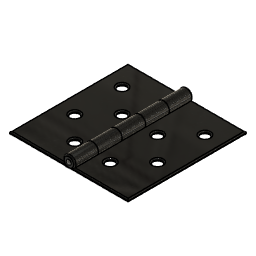
Hinge Joint (Autodesk Fusion 360 design; units mm, degrees)
Autodesk Fusion 360 part; units mm, degrees
sketch "Sketch1" plane through (0, 0, 0) normal (0, 1, 0) x (1, 0, 0)
  line L0 (0, 0) -> (50, 0)
  line L1 (50, 0) -> (50, 2.5)
  line L2 (50, 2.5) -> (0, 2.5)
  line L3 (0, 2.5) -> (0, 0)
  circle A0 centre (0, -2.5) radius 5
  circle A1 centre (0, -2.5) radius 2
  dimension "d1" = 50
  dimension "d2" = 2.5
  dimension "d3" = 10
  dimension "d4" = 4
  constraint horizontal L0
  constraint vertical L1
  constraint horizontal L2
  constraint vertical L3
  constraint coincident L0.start L3.end
  constraint coincident L2.end A0
  constraint concentric A0 A1
  measures "d1" distance of L0.start L0.end
  measures "d2" distance of L0.start L2.end
  measures "d3" diameter of A0
  measures "d4" diameter of A1
extrude "Extrude1" add sketch "Sketch1" along normal blind 100 contours L0 L1 L2 A0 makes body 1 in component "hinge1"
extrude "Extrude2" add sketch "Sketch1" along normal blind 20 contours L0 L3 A0 | L0 L3 A0 bodies 1 in component "hinge1"
pattern_linear "R-Pattern1" count 3 spacing 40 along (0, 1, 0) of "Extrude2" in component "hinge1"
extrude "Extrude1'" add sketch "Sketch1" along normal blind 100 separate body contours L0 L1 L2 A0 makes body 2 in component "hinge 2"
extrude "Extrude2'" add 1 faces at (3.5955, 20, 0.7685) along direction (0, 1, 0) blind 20 on bodies 1 bodies 2 in component "hinge 2"
extrude "Extrude3" add 1 faces at (-0.2982, 60, -1.4795) along direction (0, 1, 0) blind 20 on bodies 1 bodies 2 in component "hinge 2"
sketch "Sketch2" plane through (0, 0, 7.5) normal (0, 0, 1) x (-1, 0, 0)
  line L0 (-50, -100) -> (0, -100)
  line L1 (0, -100) -> (0, -80)
  line L2 (0, -80) -> (0, -60)
  line L3 (0, -60) -> (0, -40)
  line L4 (0, -40) -> (0, -20)
  line L5 (0, -20) -> (0, 0)
  line L6 (0, 0) -> (-50, 0)
  line L7 (-50, 0) -> (-50, -100)
  circle A0 centre (-35, -80) radius 3.75
  circle A1 centre (-35, -40) radius 3.75
  circle A2 centre (-15, -60) radius 3.75
  circle A3 centre (-15, -20) radius 3.75
  line L8 (0, 0) -> (-50, 0)
  dimension "d25" = 7.5
  dimension "d26" = 7.5
  dimension "d27" = 7.5
  dimension "d28" = 7.5
  dimension "d29" = 20
  dimension "d30" = 15
  dimension "d31" = 15
  dimension "d32" = 40
  dimension "d33" = 20
  dimension "d34" = 15
  dimension "d35" = 15
  dimension "d36" = 40
  measures "d25" diameter of A0
  measures "d26" diameter of A1
  measures "d27" diameter of A2
  measures "d28" diameter of A3
  measures "d29" distance of L0 A0.centre
  measures "d30" distance of L7 A0.centre
  measures "d31" distance of L7 A1.centre
  measures "d32" distance of A1.centre L8
  measures "d33" distance of A3.centre L8
  measures "d34" distance of L4 A3.centre
  measures "d35" distance of L1 A2.centre
  measures "d36" distance of L0 A2.centre
extrude "Extrude3'" cut sketch "Sketch2" against normal blind 50 contours A0 | A1 | A2 | A3 bodies 1 in component "hinge1"
extrude "Extrude4" cut sketch "Sketch2" against normal blind 50 contours A0 | A1 | A2 | A3 sketch seen with x (1, 0, 0) y (0, -1, 0) z (0, 0, -1) at (0, 100, 5) bodies 2 in component "hinge 2"
sketch "Sketch1 (2)" plane through (0, 0, 0) normal (0, 1, 0) x (1, 0, 0) in component "connecting rod"
  circle A0 centre (0, -2.5) radius 2
extrude "Extrude1''" add sketch "Sketch1 (2)" along normal blind 101 and the other way blind 1 separate body makes body 3 in component "connecting rod"
fillet "Fillet1" radius 2 2 edges at (-1.8647, -1, 1.7768) (-1.8647, 101, 3.2232) on bodies 3 in component "connecting rod"
fillet "Fillet1'" radius 1 16 edges at (38.4962, 78.6439, 0) (38.4962, 81.3561, -2.5) (18.4962, 58.6439, 0) (18.4962, 61.3561, -2.5) (38.4962, 38.6439, 0) (38.4962, 41.3561, -2.5) (27.1651, 0, 0) (25, 0, -2.5) (-2.5, 0, 6.8301) (18.4962, 18.6439, 0) (18.4962, 21.3561, -2.5) (50, 50, 0) (50, 50, -2.5) (27.1651, 100, 0) (25, 100, -2.5) (-2.5, 100, 6.8301) on bodies 1 in component "hinge1"
fillet "Fillet1''" radius 1 14 edges at (27.1651, 100, 0) (25, 100, -2.5) (50, 50, 0) (50, 50, -2.5) (18.4962, 78.6439, 0) (18.4962, 81.3561, -2.5) (38.4962, 58.6439, 0) (38.4962, 61.3561, -2.5) (18.4962, 38.6439, 0) (18.4962, 41.3561, -2.5) (38.4962, 18.6439, 0) (38.4962, 21.3561, -2.5) (27.1651, 0, 0) (25, 0, -2.5) on bodies 2 in component "hinge 2"
component "hinge1" placed x (1, 0, 0) y (0, 1, 0) z (0, 0, 1) at (0, 0, 0)
component "hinge 2" placed x (1, 0, 0) y (0, -1, 0) z (0, 0, -1) at (0, 100, 5)
component "connecting rod" placed x (1, 0, 0) y (0, 1, 0) z (0, 0, 1) at (0, 0, 0)
